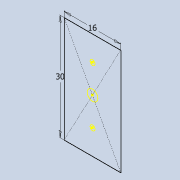
# Autodesk Inventor part: cpr_shell_1
Saved by Autodesk Inventor 2020 (Build 240168000, 168)
## iProperties
Created: 2021-10-07
Part Number: cpr_shell_1
Material: Generic
Document SubType Name: Modeling
Designer: Shuang Peng
Density: 1 g/cm^3
Appearance: Default
Author: Shuang Peng
Autodesk Inventor part; units mm, degrees
ref_plane "YZ Plane" through (0, 0, 0) normal (1, 0, 0) x (0, 1, 0)
ref_plane "XZ Plane" through (0, 0, 0) normal (0, 1, 0) x (-1, 0, 0)
ref_plane "XY Plane" through (0, 0, 0) normal (0, 0, 1) x (1, 0, 0)
ref_plane "Work Plane1" through (0, -18, -3) normal (1, 0, 0) x (0, 0, -1)
sketch "Sketch2" plane through (0, -18, -3) normal (1, 0, 0) x (0, 0, -1)
  line L0 (-2.3324, 4.2554) -> (0, 4.2554) projected
  arc A0 (-3, 4) -> (-2.3324, 4.2554) centre (-3, 5) ccw projected
  line L1 (-3, 0.5) -> (-3, 4) projected
  line L2 (0, 0.5) -> (-3, 0.5) projected
  line L3 (0, 4.2554) -> (0, 0.5) projected
  line L4 (0, 15.7446) -> (-2.3324, 15.7446) projected
  line L5 (0, 19.5) -> (0, 15.7446) projected
  line L6 (-3, 19.5) -> (0, 19.5) projected
  line L7 (-3, 16) -> (-3, 19.5) projected
  arc A1 (-2.3324, 15.7446) -> (-3, 16) centre (-3, 15) ccw projected
  line L8 (20, 4.2554) -> (22.3324, 4.2554) projected
  line L9 (20, 0.5) -> (20, 4.2554) projected
  line L10 (23, 0.5) -> (20, 0.5) projected
  line L11 (23, 4) -> (23, 0.5) projected
  arc A2 (22.3324, 4.2554) -> (23, 4) centre (23, 5) ccw projected
  line L12 (22.3324, 15.7446) -> (20, 15.7446) projected
  arc A3 (23, 16) -> (22.3324, 15.7446) centre (23, 15) ccw projected
  line L13 (23, 19.5) -> (23, 16) projected
  line L14 (20, 19.5) -> (23, 19.5) projected
  line L15 (20, 15.7446) -> (20, 19.5) projected
  line L16 (20, 4.2554) -> (20, 15.7446)
  line L17 (0, 15.7446) -> (0, 4.2554)
  line L18 (20, 10) -> (0, 10)
  line L19 (23, -10) -> (-3, -10)
  line L20 (-3, -10) -> (-3, 30)
  line L21 (-3, 30) -> (23, 30)
  line L22 (23, 30) -> (23, -10)
  line L23 (23, -10) -> (-3, 30) construction
  line L24 (-3, -10) -> (23, 30) construction
  line L25 (26, -16) -> (-6, -16)
  line L26 (-6, -16) -> (-6, 36)
  line L27 (-6, 36) -> (26, 36)
  line L28 (26, 36) -> (26, -16)
  line L29 (26, -16) -> (-6, 36) construction
  line L30 (-6, -16) -> (26, 36) construction
  point P0 (-3, 18)
  point P1 (10, 10)
  point P2 (-3, 4)
  dimension "d2" = 26
  dimension "d3" = 40
  dimension "d4" = 6
  dimension "d5" = 3
  constraints: 30 end point, 7 midpoint, 5 parallel, 4 perpendicular
  measures "d2" distance of L19.start L19.end
  measures "d3" distance of L19.end L20.end
  measures "d4" distance between parallel lines of L27 L21
  measures "d5" distance between parallel lines of L20 L26
extrude "Extrusion1" add sketch "Sketch2" along normal mid plane 4
ref_plane "Work Plane2" through (-2, -34, -13) normal (0, 0, 1) x (1, 0, 0)
sketch "Sketch3" plane through (-2, -34, 3) normal (0, 0, 1) x (1, 0, 0)
  circle A0 centre (2, 26) radius 1.5 projected
  line L0 (0, 0) -> (4, 0) projected
  line L1 (4, 52) -> (4, 0) projected
  line L2 (0, 52) -> (4, 52) projected
  line L3 (0, 0) -> (0, 52) projected
  line L4 (7, 20) -> (-3, 20)
  line L5 (-3, 20) -> (-3, 32)
  line L6 (-3, 32) -> (7, 32)
  line L7 (7, 32) -> (7, 20)
  line L8 (7, 20) -> (-3, 32) construction
  line L9 (-3, 20) -> (7, 32) construction
  point P0 (2, 34)
  point P1 (0, 20)
  point P2 (0, 32)
  dimension "d8" = 10
  dimension "d9" = 12
  constraints: 12 end point, 2 midpoint, 2 parallel, 1 horizontal, 1 perpendicular
  measures "d8" distance of L4.start L4.end
  measures "d9" distance of L4.end L5.end
extrude "Extrusion2" add sketch "Sketch3" against normal up to surface (3 mm away) contours L4 L5 L6 L3
sketch "Sketch4" plane through (-2, -34, 3) normal (0, 0, 1) x (1, 0, 0)
  circle A0 centre (2, 18) radius 0.7 projected
  circle A1 centre (2, 34) radius 0.7 projected
  circle A2 centre (2, 26) radius 1.5 projected
  line L0 (2, 26) -> (6, 26) construction
  line L1 (2, 24) -> (6, 24)
  line L2 (6, 28) -> (2, 28)
  arc A3 (2, 28) -> (2, 24) centre (2, 26) ccw
  arc A4 (6, 24) -> (6, 28) centre (6, 26) ccw
  point P0 (4, 26)
  dimension "d12" = 4
  dimension "d13" = 4
  constraints: 8 end point, 4 point on circle, 4 tangent, 2 centre point, 1 horizontal, 1 midpoint, 1 parallel
  measures "d12" distance of L0.start L0.end
  measures "d13" diameter of A4
extrude "Extrusion3" cut sketch "Sketch4" against normal blind 4 contours A0 | A1 | A2 | A3 L2 A4 L1
mirror "Mirror1" about plane through (-2, -34, -13) normal (0, 0, 1) of "Extrusion3", "Extrusion2"
body "Solid1"
